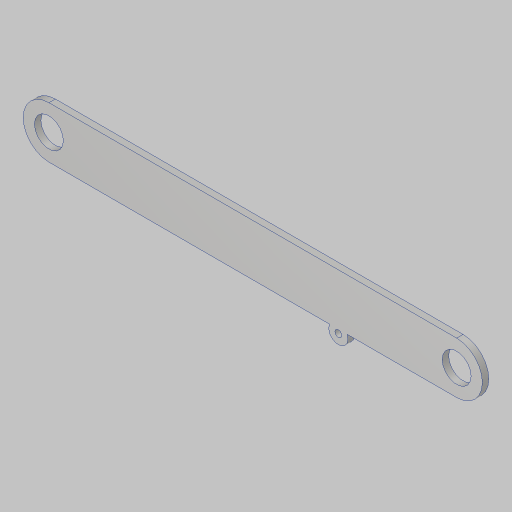
# Autodesk Inventor part: GP4-003
Saved by Autodesk Inventor 2023.5 (Build 275446000, 446)
## iProperties
Created: 2025-02-23
Part Number: GP4-003
Material: Aluminum 6061
Document SubType Name: Modeling
Designer: slick
Density: 2.7 g/cm^3
Appearance: Aluminum - Flat
Author: slick
Autodesk Inventor part; units mm, degrees
ref_plane "YZ Plane" through (0, 0, 0) normal (1, 0, 0) x (0, 1, 0)
ref_plane "XZ Plane" through (0, 0, 0) normal (0, 1, 0) x (-1, 0, 0)
ref_plane "XY Plane" through (0, 0, 0) normal (0, 0, 1) x (1, 0, 0)
sketch "Sketch1" plane through (0, 0, 0) normal (0, 0, 1) x (1, 0, 0)
  circle A0 centre (0, 0) radius 14.2875
  circle A1 centre (402.59, 0) radius 14.2875
  line L0 (0, 0) -> (402.59, 0) construction
  line L1 (0, 0) -> (402.59, 0) construction
  line L2 (402.59, 25.4) -> (0, 25.4)
  arc A2 (0, 25.4) -> (0, -25.4) centre (0, 0) ccw
  arc A3 (402.59, -25.4) -> (402.59, 25.4) centre (402.59, 0) ccw
  arc A4 (276.9873, -25.4) -> (294.5127, -25.4) centre (285.75, -29.1338) ccw
  line L3 (0, -25.4) -> (276.9873, -25.4)
  line L4 (294.5127, -25.4) -> (402.59, -25.4)
  point P0 (201.295, 0)
  dimension "d0" = 28.575
  dimension "d1" = 402.59
  dimension "d2" = 50.8
  dimension "d3" = 285.75
  dimension "d15" = 29.1338
  dimension "d16" = 19.05
  constraints: 12 end point, 6 point on circle, 6 tangent, 5 centre point, 2 coincident, 2 parallel, 1 collinear, 1 equal radius, 1 horizontal, 1 midpoint
  measures "d0" diameter of A0
  measures "d1" distance of L0.start L0.end
  measures "d2" diameter of A3
  measures "d3" horizontal distance of L0.start point (285.75, -29.134)
  measures "d15" distance from line of L0 point (285.75, -29.134)
  measures "d16" diameter of A4
extrude "Extrusion1" add sketch "Sketch1" along normal blind 6.35
hole "Hole1" at (285.75, -29.1338, 0) direction (0, 0, 1) diameter 6.7564 end through all clearance for "Flat Head Machine Screw (82)" size "1/4" standard "Ansi Unified Screw Threads"
body "Solid1"
